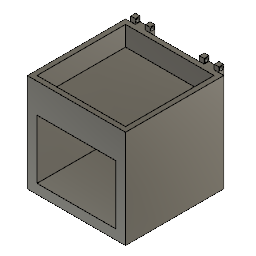
Caixa v2 (Autodesk Fusion 360 design; units mm, degrees)
Autodesk Fusion 360 part; units mm, degrees
sketch "Sketch1" plane through (0, 0, 0) normal (0, 0, 1) x (1, 0, 0)
  line L0 (50, 50) -> (-50, 50)
  line L1 (-50, 50) -> (-50, -50)
  line L2 (-50, -50) -> (50, -50)
  line L3 (50, -50) -> (50, 50)
  line L4 (50, 50) -> (-50, -50) construction
  line L5 (-50, 50) -> (50, -50) construction
  dimension "d1" = 100
  dimension "d2" = 100
  constraint horizontal L0
  constraint perpendicular L0 L1
  constraint parallel L0 L2
  constraint parallel L1 L3
  constraint coincident L4 origin
  constraint coincident L5 origin
  measures "d1" distance of L1.end L2.end
  measures "d2" distance of L0.end L1.end
extrude "Extrude1" add sketch "Sketch1" along normal blind 100
sketch "Sketch2" plane through (0, 0, 100) normal (0, 0, 1) x (-1, 0, 0)
  line L0 (-50, 50) -> (-50, -50)
  line L1 (-50, -50) -> (50, -50)
  line L2 (50, -50) -> (50, 50)
  line L3 (50, 50) -> (-50, 50)
  line L4 (-45, -45) -> (45, -45)
  line L5 (45, -45) -> (45, 45)
  line L6 (45, 45) -> (-45, 45)
  line L7 (-45, 45) -> (-45, -45)
  line L8 (-45, -45) -> (45, 45) construction
  line L9 (45, -45) -> (-45, 45) construction
  dimension "d6" = 90
  dimension "d7" = 90
  constraint horizontal L4
  constraint perpendicular L4 L5
  constraint parallel L4 L6
  constraint parallel L5 L7
  constraint coincident L8 origin
  constraint coincident L9 origin
  measures "d6" distance of L5.end L6.end
  measures "d7" distance of L4.end L5.end
extrude "Extrude2" cut sketch "Sketch2" against normal blind 20 contours L4 L5 L6 L7
sketch "Sketch3" plane through (0, -50, 0) normal (0, -1, 0) x (1, 0, 0)
  line L0 (-50, 0) -> (50, 0)
  line L1 (50, 0) -> (50, 100)
  line L2 (50, 100) -> (-50, 100)
  line L3 (-50, 100) -> (-50, 0)
  line L4 (-40, 10) -> (-40, 40)
  line L5 (-40, 40) -> (40, 40)
  line L6 (40, 40) -> (40, 10)
  line L7 (40, 10) -> (-40, 10)
  line L8 (-40, 70) -> (40, 70)
  line L9 (40, 70) -> (40, 40)
  line L10 (-40, 40) -> (-40, 70)
  constraint vertical L4
  constraint perpendicular L4 L5
  constraint perpendicular L5 L6
  constraint perpendicular L4 L7
  constraint perpendicular L4 L8
  constraint perpendicular L5 L9
  constraint perpendicular L8 L10
extrude "Extrude3" cut sketch "Sketch3" against normal blind 90 contours L4 L5 L6 L7 | L5 L8 L9 L10
sketch "Sketch4" plane through (0, 0, 100) normal (0, 0, 1) x (-1, 0, 0)
  line L0 (45, -45) -> (-45, -45)
  line L1 (-45, -45) -> (-45, 45)
  line L2 (-45, 45) -> (45, 45)
  line L3 (45, 45) -> (45, -45)
  line L4 (-50, 50) -> (-50, -50)
  line L5 (-50, -50) -> (50, -50)
  line L6 (50, -50) -> (50, 50)
  line L7 (50, 50) -> (-50, 50)
  line L8 (45, -50) -> (45, -55)
  line L9 (-45, -50) -> (-45, -55)
  line L10 (-45, -55) -> (-25, -55)
  line L11 (-25, -55) -> (-25, -50)
  line L12 (45, -55) -> (25, -55)
  line L13 (25, -55) -> (25, -50)
  dimension "d12" = 5
  dimension "d13" = 5
  dimension "d14" = 20
  dimension "d15" = 20
  constraint coincident L5 L8.start
  constraint perpendicular L5 L8
  constraint coincident L5 L9.start
  constraint perpendicular L5 L9
  constraint perpendicular L9 L10
  constraint coincident L5 L11.end
  constraint perpendicular L5 L11
  constraint perpendicular L8 L12
  constraint coincident L5 L13.end
  constraint perpendicular L5 L13
  measures "d12" distance of L8.start L8.end
  measures "d13" distance of L9.start L9.end
  measures "d14" distance of L9.end L10.end
  measures "d15" distance of L8.end L12.end
extrude "Extrude4" add sketch "Sketch4" along normal mid plane 10 contours L5 L9 L10 L11 | L5 L8 L12 L13
sketch "Sketch5" plane through (0, 0, 105) normal (0, 0, 1) x (-1, 0, 0)
  line L0 (-45, -50) -> (-45, -55)
  line L1 (-45, -55) -> (-25, -55)
  line L2 (-25, -55) -> (-25, -50)
  line L3 (-25, -50) -> (-45, -50)
  line L4 (-25, -55) -> (-30, -55)
  line L5 (-30, -55) -> (-40, -55)
  line L6 (-40, -55) -> (-40, -50)
  line L7 (-30, -50) -> (-30, -55)
  line L8 (25, -55) -> (30, -55)
  line L9 (30, -55) -> (40, -55)
  line L10 (40, -55) -> (40, -50)
  line L11 (40, -50) -> (30, -50)
  line L12 (30, -50) -> (30, -55)
  constraint coincident L1.end L2.start
  constraint coincident L1 L4.end
  constraint perpendicular L2 L4
  constraint coincident L1 L5.end
  constraint perpendicular L2 L5
  constraint coincident L3 L6.end
  constraint perpendicular L3 L6
  constraint coincident L3 L7.start
  constraint perpendicular L4 L7
  constraint horizontal L8
  constraint parallel L8 L9
  constraint perpendicular L9 L10
  constraint perpendicular L10 L11
  constraint perpendicular L9 L12
extrude "Extrude5" cut sketch "Sketch5" against normal blind 5 contours L1 L3 L5 L6 L7 | L9 L10 L11 L12
sketch "Sketch9" plane through (45, 0, 0) normal (1, 0, 0) x (0, 1, 0)
  line L0 (55, 95) -> (55, 105)
  line L1 (55, 105) -> (50, 105)
  line L2 (50, 105) -> (50, 100)
  line L3 (50, 100) -> (50, 95)
  line L4 (50, 95) -> (55, 95)
  circle A0 centre (52.5, 102.5) radius 2
extrude "Extrude7" cut sketch "Sketch9" against normal blind 130 contours A0
